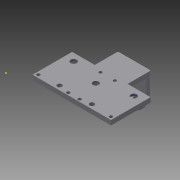
# Autodesk Inventor part: double-right2.0
Saved by Autodesk Inventor 2014 (Build 180170000, 170)
## iProperties
Created: 2013-11-04
Part Number: double-right2.0
Material: Generic
Document SubType Name: Modeling
Designer: stephen
Density: 1 g/cm^3
Appearance: Default
Author: stephen
Autodesk Inventor part; units mm, degrees
ref_plane "YZ Plane" through (0, 0, 0) normal (1, 0, 0) x (0, 1, 0)
ref_plane "XZ Plane" through (0, 0, 0) normal (0, 1, 0) x (-1, 0, 0)
ref_plane "XY Plane" through (0, 0, 0) normal (0, 0, 1) x (1, 0, 0)
sketch "Sketch1" plane through (0, 0, 0) normal (0, 0, 1) x (1, 0, 0)
  circle A0 centre (120.6347, 53.34) radius 4.15
  circle A1 centre (87.3962, 12.795) radius 2.2225
  circle A2 centre (101.7312, 15.24) radius 3.175
  circle A3 centre (79.6967, 42.545) radius 4.15
  circle A4 centre (89.5011, 58.7375) radius 2.0955
  circle A5 centre (38.7587, 53.34) radius 4.15
  circle A6 centre (57.6622, 15.24) radius 3.175
  circle A7 centre (71.9972, 12.795) radius 2.2225
  circle A8 centre (69.8923, 58.7375) radius 2.0955
  line L0 (130.6347, 53.34) -> (133.4205, 53.34)
  line L1 (79.6967, 42.545) -> (77.0905, 39.3154)
  line L2 (133.4205, 14.5) -> (133.4205, 63.5)
  line L3 (130.6347, 53.34) -> (120.6347, 53.34)
  line L4 (79.6967, 42.545) -> (83.0499, 40.1)
  line L5 (102.0937, 89.1573) -> (102.0937, 63.5)
  line L6 (57.2997, 89.1573) -> (57.2997, 63.5)
  line L7 (133.4205, 63.5) -> (102.0937, 63.5)
  line L8 (57.2997, 63.5) -> (27.7457, 63.5)
  line L9 (27.7457, 63.5) -> (57.2997, 63.5)
  line L10 (102.0937, 63.5) -> (133.4205, 63.5)
  line L11 (133.4205, 63.5) -> (102.0937, 63.5)
  line L12 (57.2997, 63.5) -> (27.7457, 63.5)
  line L13 (27.7457, 63.5) -> (57.2997, 63.5)
  line L14 (102.0937, 63.5) -> (133.4205, 63.5)
  line L15 (27.7457, 63.5) -> (57.2997, 63.5)
  line L16 (102.0937, 63.5) -> (133.4205, 63.5)
  line L17 (27.7457, 63.5) -> (57.2997, 63.5)
  line L18 (102.0937, 63.5) -> (133.4205, 63.5)
  line L19 (133.4205, 63.5) -> (102.0937, 63.5)
  line L20 (57.2997, 63.5) -> (27.7457, 63.5)
  line L21 (27.7457, 63.5) -> (57.2997, 63.5)
  line L22 (102.0937, 63.5) -> (133.4205, 63.5)
  line L23 (27.7457, 21.8733) -> (27.7457, 14.5)
  line L24 (57.2997, 89.1573) -> (57.2997, 95.1573)
  line L25 (57.2997, 95.1573) -> (102.0937, 95.1573)
  line L26 (102.0937, 95.1573) -> (102.0937, 89.1573)
  line L27 (27.7457, 14.5) -> (26.4727, 14.5)
  line L28 (26.4727, 14.5) -> (26.4727, 63.5)
  line L29 (26.4727, 63.5) -> (27.7457, 63.5)
  circle A9 centre (79.6967, 42.545) radius 35.0868
  line L30 (67.8053, 9.5347) -> (57.6622, 15.24)
  line L31 (57.6622, 15.24) -> (57.2997, 15.6892)
  line L32 (67.8053, 9.5347) -> (79.6967, 9.5347) construction
  line L33 (101.7312, 15.24) -> (108.0474, 15.24) construction
  line L34 (26.4727, 14.5) -> (26.4727, 9.5)
  line L35 (26.4727, 9.5) -> (133.4205, 9.5)
  line L36 (133.4205, 9.5) -> (133.4205, 14.5)
  line L37 (88.3962, 12.795) -> (87.3962, 12.795)
  line L38 (70.9972, 12.795) -> (71.9972, 12.795)
  line L39 (93.3492, 58.7375) -> (91.3492, 58.7375)
  line L40 (66.0442, 58.7375) -> (68.0442, 58.7375)
  circle A10 centre (31.4727, 14.5) radius 2.2225
  line L41 (79.6967, 42.545) -> (79.6967, 65.8401)
  point P0 (0, 0)
  point P1 (-18.1648, 53.34)
  point P2 (27.7457, 53.34)
  dimension "d0" = 8.3
  dimension "d44" = 10
  dimension "d91" = 1.273
  dimension "d93" = 5
  dimension "d102" = 4.7625
  dimension "d103" = 8.3
  dimension "d104" = 1
  dimension "d105" = 1
  dimension "d106" = 2
  dimension "d107" = 2
  dimension "d108" = 5
  dimension "d109" = 5
  dimension "d119" = 9.8044
  dimension "d120" = 9.8044
  constraints: 84 end point, 11 centre point, 10 horizontal, 9 perpendicular, 5 point on circle, 4 point on line, 2 collinear, 2 parallel, 1 coincident
  measures "d0" diameter of A0
  measures "d44" distance of L3.start L3.end
  measures "d91" distance of L23.end L27.end
  measures "d93" distance of L27.end L34.end
  measures "d102" distance from line of A8.centre L8
  measures "d103" diameter of A5
  measures "d104" distance of L37.start L37.end
  measures "d105" distance of L38.start L38.end
  measures "d106" distance of L39.start L39.end
  measures "d107" distance of L40.start L40.end
  measures "d108" distance from line of L34 A10.centre
  measures "d109" distance from line of L35 A10.centre
  measures "d119" distance from line of L41 A4.centre
  measures "d120" distance from line of L41 A8.centre
extrude "Extrusion1" add sketch "Sketch1" along normal blind 6.35 contours A2 A9 L7 L2 L36 L35 | A2 A9 L35 L30 A6 L8 L6 L5 L7 | L35 L34 L28 L29 L8 A9 A6 | A9 L6 L24 L25 L26 L5 | A9 A6 L30 | A9 L30 A6 | L1 L4 A3 | A3 L41 L1 | L4 L41 A3 | A10 picked at (64.4705, 11.2739) picked at (58.8626, 14.5037)
sketch "Sketch3" plane through (0, 0, 0) normal (0, 0, -1) x (-1, 0, 0)
  circle A0 centre (-79.6967, 42.545) radius 4 projected
  circle A1 centre (-79.6967, 42.545) radius 11.15
  circle A2 centre (-79.6967, 42.545) radius 12.5
  point P0 (0, 0)
  dimension "d6" = 22.3
  dimension "d7" = 25
  constraints: 2 centre point, 2 coincident
  measures "d6" diameter of A1
  measures "d7" diameter of A2
extrude "Extrusion2" add sketch "Sketch3" along normal blind 2 contours A2
sketch "Sketch4" plane through (0, 0, 0) normal (0, 0, -1) x (-1, 0, 0)
  line L0 (-57.2997, 63.5) -> (-26.4727, 63.5) projected
  circle A0 centre (-120.6347, 53.34) radius 4.15 projected
  arc A1 (-125.2278, 63.5) -> (-116.0415, 63.5) centre (-120.6347, 53.34) ccw
  arc A2 (-127.9164, 63.5) -> (-113.3529, 63.5) centre (-120.6347, 53.34) ccw
  line L1 (-133.4205, 63.5) -> (-102.0937, 63.5) projected
  line L2 (-26.4727, 14.5) -> (-133.4205, 14.5) projected
  line L3 (-127.9164, 63.5) -> (-125.2278, 63.5)
  line L4 (-116.0415, 63.5) -> (-113.3529, 63.5)
  point P0 (18.1648, 63.5)
  point P1 (-143.4205, 63.5)
  point P2 (0, 0)
  point P3 (-27.7457, 63.5)
  point P4 (-27.7457, 14.5)
  dimension "d10" = 22.3
  dimension "d11" = 25
  constraints: 4 end point, 4 point on circle, 2 centre point, 2 coincident, 1 collinear, 1 parallel, 5 other
  measures "d10" diameter of A1
  measures "d11" diameter of A2
extrude "Extrusion16" add sketch "Sketch4" along normal blind 2 contours A1 L1 A2
sketch "Sketch5" plane through (0, 0, 0) normal (0, 0, -1) x (-1, 0, 0)
  line L0 (-57.2997, 63.5) -> (-26.4727, 63.5) projected
  circle A0 centre (-38.7587, 53.34) radius 4.15 projected
  arc A1 (-43.3518, 63.5) -> (-34.1655, 63.5) centre (-38.7587, 53.34) ccw
  arc A2 (-46.0404, 63.5) -> (-31.4769, 63.5) centre (-38.7587, 53.34) ccw
  point P0 (18.1648, 63.5)
  point P1 (0, 0)
  point P2 (-27.7457, 63.5)
  dimension "d14" = 22.3
  dimension "d15" = 25
  constraints: 4 point on circle, 4 point on line, 2 centre point, 2 coincident
  measures "d14" diameter of A1
  measures "d15" diameter of A2
extrude "Extrusion4" add sketch "Sketch5" along normal blind 2 contours L0 A1 A2
sketch "Sketch6" plane through (0, 0, 0) normal (0, 0, -1) x (-1, 0, 0)
  circle A0 centre (-120.6347, 53.34) radius 4.15 projected
  arc A1 (-124.8506, 63.5) -> (-116.4187, 63.5) centre (-120.6347, 53.34) ccw projected
  line L0 (-27.7457, 63.5) -> (-27.7457, 59.253) projected
  line L1 (-124.8506, 63.5) -> (-116.4187, 63.5)
  arc A2 (-124.8506, 63.5) -> (-116.4187, 63.5) centre (-120.6347, 53.34) ccw
  point P0 (0, 0)
  constraints: 2 end point, 2 point on circle, 1 centre point, 1 coincident, 1 perpendicular
sketch "Sketch7" plane through (0, 0, 0) normal (0, 0, -1) x (-1, 0, 0)
  arc A0 (-43.3518, 63.5) -> (-34.1655, 63.5) centre (-38.7587, 53.34) ccw projected
  line L0 (-43.3518, 63.5) -> (-34.1655, 63.5) projected
  circle A1 centre (-38.7587, 53.34) radius 4.15 projected
  point P0 (0, 0)
extrude "Extrusion6" cut sketch "Sketch7" against normal blind 5
sketch "Sketch8" plane through (79.6967, 42.545, 0) normal (0, 0, -1) x (-1, 0, 0)
  circle A0 centre (0, 0) radius 11.15 projected
  circle A1 centre (0, 0) radius 4 projected
  point P0 (79.6967, -42.545)
extrude "Extrusion7" cut sketch "Sketch8" against normal blind 5
sketch "Sketch9" plane through (0, 0, 0) normal (0, 0, -1) x (-1, 0, 0)
  line L0 (-57.2997, 95.1573) -> (-57.2997, 63.5) projected
  line L1 (-102.0937, 95.1573) -> (-57.2997, 95.1573)
  line L2 (-57.2997, 95.1573) -> (-57.2997, 89.1573)
  line L3 (-57.2997, 89.1573) -> (-102.0937, 89.1573)
  line L4 (-102.0937, 89.1573) -> (-102.0937, 95.1573)
  point P0 (0, 0)
  dimension "d49" = 6
  constraints: 8 end point, 2 parallel, 1 horizontal, 1 perpendicular, 1 point on line
  measures "d49" distance of L1.end L2.end
extrude "Extrusion8" add sketch "Sketch9" along normal blind 21.5
sketch "Sketch10" plane through (0, 0, -21.5) normal (0, 0, -1) x (-1, 0, 0)
  line L0 (-57.2997, 89.1573) -> (-57.2997, 95.1573) projected
  line L1 (-57.2997, 95.1573) -> (-102.0937, 95.1573) projected
  line L2 (-102.0937, 95.1573) -> (-102.0937, 89.1573) projected
  line L3 (-102.0937, 89.1573) -> (-57.2997, 89.1573) projected
  line L4 (-102.0937, 95.1573) -> (-57.2997, 95.1573)
  line L5 (-57.2997, 95.1573) -> (-57.2997, 51.4211)
  line L6 (-102.0937, 51.4211) -> (-102.0937, 95.1573)
  line L7 (-93.5397, 87.9742) -> (-93.5397, 79.7192)
  line L8 (-96.7147, 79.7192) -> (-96.7147, 87.9742)
  arc A0 (-96.7147, 79.7192) -> (-93.5397, 79.7192) centre (-95.1272, 79.7192) ccw
  arc A1 (-82.8717, 79.4017) -> (-88.1607, 58.5161) centre (-82.8717, 68.2892) ccw
  line L9 (-82.8717, 79.4017) -> (-76.5217, 79.4017)
  line L10 (-96.7147, 48.7312) -> (-96.7147, 56.9862)
  arc A2 (-93.5397, 56.9862) -> (-96.7147, 56.9862) centre (-95.1272, 56.9862) ccw
  line L11 (-93.5397, 56.9862) -> (-93.5397, 48.7312)
  arc A3 (-62.5517, 56.9862) -> (-65.7267, 56.9862) centre (-64.1392, 56.9862) ccw
  arc A4 (-71.2327, 58.5161) -> (-76.5217, 79.4017) centre (-76.5217, 68.2892) ccw
  line L12 (-65.7267, 48.7312) -> (-65.7267, 56.9862)
  line L13 (-62.5517, 56.9862) -> (-62.5517, 48.7312)
  line L14 (-65.7267, 79.7192) -> (-65.7267, 87.9742)
  line L15 (-62.5517, 87.9742) -> (-62.5517, 79.7192)
  arc A5 (-65.7267, 79.7192) -> (-62.5517, 79.7192) centre (-64.1392, 79.7192) ccw
  line L16 (-79.6967, 57.1767) -> (-79.6967, 57.6399)
  line L17 (-79.6967, 57.1767) -> (-79.6967, 57.6399)
  line L18 (-102.0937, 89.1573) -> (-102.0937, 51.4211)
  line L19 (-88.1607, 51.4211) -> (-88.1607, 51.4211)
  line L20 (-71.2327, 58.5161) -> (-71.2327, 51.4211)
  line L21 (-71.2327, 51.4211) -> (-71.2327, 51.4211)
  line L22 (-61.2997, 47.4211) -> (-67.2327, 47.4211)
  line L23 (-92.1607, 47.4211) -> (-98.0937, 47.4211)
  line L24 (-88.1607, 58.5161) -> (-88.1607, 51.4211)
  line L25 (-88.1607, 79.4017) -> (-88.1607, 78.0623)
  arc A6 (-92.1607, 47.4211) -> (-88.1607, 51.4211) centre (-92.1607, 51.4211) ccw
  arc A7 (-71.2327, 51.4211) -> (-67.2327, 47.4211) centre (-67.2327, 51.4211) ccw
  line L26 (-95.1272, 87.9742) -> (-95.1272, 79.7192) construction
  line L27 (-96.7147, 87.9742) -> (-96.7147, 79.7192)
  line L28 (-93.5397, 79.7192) -> (-93.5397, 87.9742)
  arc A8 (-96.7147, 79.7192) -> (-93.5397, 79.7192) centre (-95.1272, 79.7192) ccw
  line L29 (-64.1392, 79.7192) -> (-64.1392, 87.9742) construction
  line L30 (-65.7267, 79.7192) -> (-65.7267, 87.9742)
  line L31 (-62.5517, 87.9742) -> (-62.5517, 79.7192)
  arc A9 (-65.7267, 79.7192) -> (-62.5517, 79.7192) centre (-64.1392, 79.7192) ccw
  line L32 (-64.1392, 48.7312) -> (-64.1392, 56.9862) construction
  line L33 (-65.7267, 48.7312) -> (-65.7267, 56.9862)
  line L34 (-62.5517, 56.9862) -> (-62.5517, 48.7312)
  arc A10 (-62.5517, 56.9862) -> (-65.7267, 56.9862) centre (-64.1392, 56.9862) ccw
  line L35 (-95.1272, 48.7312) -> (-95.1272, 56.9862) construction
  line L36 (-96.7147, 48.7312) -> (-96.7147, 56.9862)
  line L37 (-93.5397, 56.9862) -> (-93.5397, 48.7312)
  arc A11 (-93.5397, 56.9862) -> (-96.7147, 56.9862) centre (-95.1272, 56.9862) ccw
  line L38 (-102.0937, 51.4211) -> (-102.0937, 47.4211)
  line L39 (-98.0937, 47.4211) -> (-102.0937, 47.4211)
  line L40 (-57.2997, 51.4211) -> (-57.2997, 47.4211)
  line L41 (-61.2997, 47.4211) -> (-57.2997, 47.4211)
  line L42 (-57.2997, 89.1573) -> (-102.0937, 89.1573)
  arc A12 (-62.5517, 87.9742) -> (-63.0807, 89.1573) centre (-64.1392, 87.9742) ccw
  arc A13 (-65.1976, 89.1573) -> (-65.7267, 87.9742) centre (-64.1392, 87.9742) ccw
  arc A14 (-62.5517, 87.9742) -> (-63.0807, 89.1573) centre (-64.1392, 87.9742) ccw
  arc A15 (-65.1976, 89.1573) -> (-65.7267, 87.9742) centre (-64.1392, 87.9742) ccw
  arc A16 (-93.5397, 87.9742) -> (-94.0687, 89.1573) centre (-95.1272, 87.9742) ccw
  arc A17 (-96.1856, 89.1573) -> (-96.7147, 87.9742) centre (-95.1272, 87.9742) ccw
  arc A18 (-93.5397, 87.9742) -> (-94.0687, 89.1573) centre (-95.1272, 87.9742) ccw
  arc A19 (-96.1856, 89.1573) -> (-96.7147, 87.9742) centre (-95.1272, 87.9742) ccw
  arc A20 (-65.7267, 48.7312) -> (-65.0357, 47.4211) centre (-64.1392, 48.7312) ccw
  arc A21 (-63.2426, 47.4211) -> (-62.5517, 48.7312) centre (-64.1392, 48.7312) ccw
  arc A22 (-65.7267, 48.7312) -> (-65.0357, 47.4211) centre (-64.1392, 48.7312) ccw
  arc A23 (-63.2426, 47.4211) -> (-62.5517, 48.7312) centre (-64.1392, 48.7312) ccw
  arc A24 (-96.7147, 48.7312) -> (-96.0237, 47.4211) centre (-95.1272, 48.7312) ccw
  arc A25 (-94.2306, 47.4211) -> (-93.5397, 48.7312) centre (-95.1272, 48.7312) ccw
  arc A26 (-96.7147, 48.7312) -> (-96.0237, 47.4211) centre (-95.1272, 48.7312) ccw
  arc A27 (-94.2306, 47.4211) -> (-93.5397, 48.7312) centre (-95.1272, 48.7312) ccw
  point P0 (0, 0)
  point P1 (-71.2327, 47.4211)
  point P2 (-88.1607, 47.4211)
  point P3 (-95.1272, 83.8467)
  point P4 (-64.1392, 83.8467)
  point P5 (-64.1392, 52.8587)
  point P6 (-95.1272, 52.8587)
  dimension "d60" = 4
  constraints: 86 end point, 58 point on circle, 28 centre point, 20 tangent, 15 point on line, 9 parallel, 6 perpendicular, 4 midpoint, 2 collinear, 2 symmetric about line, 1 equal radius, 1 horizontal
  measures "d60" radius of A6
extrude "Extrusion20" add sketch "Sketch10" along normal blind 6 contours L5 L40 L41 L22 A21 L13 A3 L12 A20 A7 L20 A4 L9 A1 L24 A6 L23 A25 L11 A2 L10 A24 L39 L38 L6 L3 A17 L8 A0 L7 A16 A13 L14 A5 L15 A12
sketch "Sketch12" plane through (0, 0, -21.5) normal (0, 0, -1) x (-1, 0, 0)
  line L0 (-57.2997, 89.1573) -> (-57.2997, 95.1573) projected
  line L1 (-57.2997, 95.1573) -> (-102.0937, 95.1573) projected
  line L2 (-102.0937, 95.1573) -> (-102.0937, 89.1573) projected
  line L3 (-102.0937, 89.1573) -> (-57.2997, 89.1573) projected
  point P0 (0, 0)
extrude "Extrusion12" add sketch "Sketch12" along normal blind 6
sketch "Sketch15" plane through (0, 0, 0) normal (0, 0, -1) x (-1, 0, 0)
  line L0 (-102.0937, 63.5) -> (-105.0937, 63.5)
  line L1 (-108.0937, 63.5) -> (-108.0937, 47.427)
  line L2 (-108.0937, 47.427) -> (-104.0937, 47.427)
  line L3 (-104.0937, 47.427) -> (-104.0937, 63.5)
  line L4 (-31.4769, 63.5) -> (-26.4727, 63.5) projected
  line L5 (-105.0937, 63.5) -> (-107.0937, 63.5)
  line L6 (-104.0937, 47.427) -> (-107.0937, 47.427)
  line L7 (-107.0937, 63.5) -> (-104.0937, 63.5)
  line L8 (-104.0937, 63.5) -> (-104.0937, 47.427)
  line L9 (-108.0937, 63.5) -> (-104.0937, 63.5)
  line L10 (-104.0937, 63.5) -> (-104.0937, 47.427)
  line L11 (-104.0937, 47.427) -> (-108.0937, 47.427)
  line L12 (-108.0937, 47.427) -> (-108.0937, 63.5)
  point P0 (0, 0)
  dimension "d121" = 2
  dimension "d123" = 16.073
  constraints: 24 end point, 5 parallel, 3 horizontal, 2 perpendicular, 1 collinear
  measures "d121" distance of L5.start L5.end
  measures "d123" distance of L3.end L2.end
extrude "Extrusion13" add sketch "Sketch15" along normal blind 27.5
sketch "Sketch17" plane through (0, 0, 0) normal (0, 0, -1) x (-1, 0, 0)
  line L0 (-57.2997, 63.5) -> (-46.0404, 63.5) projected
  line L1 (-57.2997, 47.427) -> (-53.2997, 47.427)
  line L2 (-52.2997, 47.427) -> (-52.2997, 63.5)
  line L3 (-53.2997, 63.5) -> (-57.2997, 63.5)
  line L4 (-56.2997, 63.5) -> (-56.2997, 47.427)
  line L5 (-53.2997, 63.5) -> (-52.2997, 63.5)
  line L6 (-56.2997, 63.5) -> (-52.2997, 63.5)
  line L7 (-52.2997, 63.5) -> (-52.2997, 47.427)
  line L8 (-52.2997, 47.427) -> (-56.2997, 47.427)
  line L9 (-56.2997, 47.427) -> (-56.2997, 63.5)
  point P0 (0, 0)
  dimension "d76" = 4
  dimension "d122" = 1
  constraints: 18 end point, 4 parallel, 2 horizontal, 2 perpendicular, 1 point on line
  measures "d76" distance of L3.start L3.end
  measures "d122" distance of L5.start L5.end
extrude "Extrusion15" add sketch "Sketch17" along normal blind 27.5
sketch "Sketch18" plane through (79.6967, 42.545, 0) normal (0, 0, -1) x (-1, 0, 0)
  circle A0 centre (0, 0) radius 4 projected
  point P0 (79.6967, -42.545)
extrude "Extrusion18" cut sketch "Sketch18" against normal blind 10
sketch "Sketch19" plane through (0, 0, 0) normal (0, 0, -1) x (-1, 0, 0)
  arc A0 (-125.2278, 63.5) -> (-116.0415, 63.5) centre (-120.6347, 53.34) ccw projected
  line L0 (-125.2278, 63.5) -> (-116.0415, 63.5) projected
  circle A1 centre (-120.6347, 53.34) radius 4.15 projected
  point P0 (0, 0)
extrude "Extrusion19" cut sketch "Sketch19" against normal blind 5
sketch "Sketch22" plane through (0, 0, 6.35) normal (0, 0, 1) x (1, 0, 0)
  line L0 (26.4727, 63.5) -> (26.4727, 9.5) projected
  line L1 (26.4727, 9.5) -> (133.4205, 9.5) projected
  circle A0 centre (30.4727, 13.5) radius 2.2225
  point P0 (0, 0)
  dimension "d110" = 4
  dimension "d111" = 4
  constraints: 1 centre point
  measures "d110" distance from line of L0 A0.centre
  measures "d111" distance from line of L1 A0.centre
extrude "Extrusion23" cut sketch "Sketch22" against normal through all
sketch "Sketch23" plane through (0, 0, 6.35) normal (0, 0, 1) x (1, 0, 0)
  circle A0 centre (30.4727, 13.5) radius 2.2225 projected
  line L0 (26.4727, 9.5) -> (133.4205, 9.5) projected
  line L1 (133.4205, 9.5) -> (133.4205, 63.5) projected
  circle A1 centre (129.4205, 13.5) radius 2.2225
  point P0 (0, 0)
  dimension "d114" = 4
  dimension "d115" = 4
  dimension "d116" = 98.9478
  constraints: 1 centre point
  measures "d114" distance from line of A1.centre L1
  measures "d115" distance from line of L0 A1.centre
  measures "d116" distance of A0.centre A1.centre
extrude "Extrusion24" cut sketch "Sketch23" against normal through all contours A1
sketch "Sketch24" plane through (102.0937, 63.5, 6.35) normal (1, 0, 0) x (0, 0, -1)
  line L0 (27.85, 25.6573) -> (27.85, -16.0789) projected
  line L1 (33.85, -16.0789) -> (27.85, -16.0789)
  line L2 (27.85, -16.0789) -> (27.85, 0)
  line L3 (27.85, 0) -> (33.85, 0)
  line L4 (33.85, 0) -> (33.85, -16.0789)
  point P0 (6.35, -63.5)
  constraints: 8 end point, 2 parallel, 1 horizontal, 1 perpendicular, 1 point on line
extrude "Extrusion25" add sketch "Sketch24" along normal blind 2
sketch "Sketch25" plane through (57.2997, 63.5, 6.35) normal (-1, 0, 0) x (0, 0, 1)
  line L0 (-27.85, -16.0789) -> (-27.85, 25.6573) projected
  line L1 (-33.85, -16.0789) -> (-27.85, -16.0789)
  line L2 (-27.85, -16.0789) -> (-27.85, 0)
  line L3 (-27.85, 0) -> (-33.85, 0)
  line L4 (-33.85, 0) -> (-33.85, -16.0789)
  point P0 (-6.35, -63.5)
  constraints: 8 end point, 2 parallel, 1 horizontal, 1 perpendicular, 1 point on line
extrude "Extrusion26" add sketch "Sketch25" along normal blind 2
fillet "Fillet5" radius 2 14 edges at (52.2997, 55.4635, -27.5) (52.2997, 47.427, -13.75) (59.2711, 47.4211, -27.5) (70.0611, 48.5927, -27.5) (71.2327, 54.9686, -27.5) (66.1342, 47.4211, -27.5) (88.1607, 54.9686, -27.5) (93.1956, 47.4211, -27.5) (89.3322, 48.5927, -27.5) (100.0587, 47.4211, -27.5) (108.0937, 47.427, -13.75) (57.2997, 79.3287, -27.5) (108.0937, 55.4635, -27.5) (102.0937, 79.3287, -27.5)
fillet "Fillet6" radius 2 5 edges at (101.5079, 95.1573, -26.9142) (102.0937, 95.1573, -9.575) (57.8854, 95.1573, -26.9142) (57.2997, 95.1573, -9.575) (79.6967, 95.1573, -27.5)
body "Solid1"
